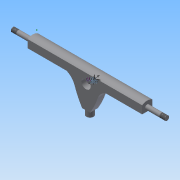
# Autodesk Inventor part: Truck
Saved by Autodesk Inventor 2015 (Build 190159000, 159)
## iProperties
Created: 2015-11-29
Part Number: Truck
Material: Generic
Document SubType Name: Modeling
Designer: JoshuaYuan
Density: 1 g/cm^3
Appearance: Default
Author: JoshuaYuan
Autodesk Inventor part; units mm, degrees
ref_plane "YZ Plane" through (0, 0, 0) normal (1, 0, 0) x (0, 1, 0)
ref_plane "XZ Plane" through (0, 0, 0) normal (0, 1, 0) x (-1, 0, 0)
ref_plane "XY Plane" through (0, 0, 0) normal (0, 0, 1) x (1, 0, 0)
sketch "Sketch1" plane through (0, 0, 0) normal (1, 0, 0) x (0, 1, 0)
  line L0 (-6.1783, -17.5347) -> (-20.1483, -17.5347)
  line L1 (-20.1483, -17.5347) -> (-20.1483, -35.5687)
  line L2 (-20.1483, -35.5687) -> (-6.1783, -35.5687)
  arc A0 (-6.1783, -35.5687) -> (-6.1783, -17.5347) centre (-19.1426, -26.5517) ccw
  point P0 (0, 0)
  dimension "d0" = 13.97
  dimension "d1" = 18.034
  constraints: 6 end point, 2 perpendicular, 2 point on circle, 1 centre point, 1 horizontal, 1 parallel
  measures "d0" distance of L1.end L2.end
  measures "d1" distance of L0.end L1.end
extrude "Truck Axle" add sketch "Sketch1" along normal blind 203.2
sketch "Sketch2" plane through (203.2, 0, 0) normal (1, 0, 0) x (0, 0, -1)
  circle A0 centre (26.5517, -13.1633) radius 3.9688
  line L0 (17.5347, -6.1783) -> (17.5347, -20.1483) projected
  line L1 (17.5347, -13.1633) -> (35.5687, -13.1633) construction
  line L2 (35.5687, -20.1483) -> (35.5687, -6.1783) projected
  point P0 (0, 0)
  point P1 (26.5517, -13.1633)
  dimension "d40" = 7.9375
  constraints: 3 midpoint, 2 end point, 1 centre point, 1 coincident
  measures "d40" diameter of A0
extrude "Axle" add sketch "Sketch2" along normal blind 34.925
ref_plane "Work Plane1" through (101.6, 0, 0) normal (1, 0, 0) x (0, 0, -1)
mirror "Other Axle" about plane through (101.6, 0, 0) normal (1, 0, 0) of "Axle"
ref_plane "Work Plane3" through (0, -20.1483, -26.5517) normal (0, 0, 1) x (1, 0, 0)
sketch "Sketch4" plane through (0, -20.1483, -26.5517) normal (0, 0, 1) x (1, 0, 0)
  line L0 (0, 0) -> (203.2, 0) projected
  line L1 (94.615, -45.72) -> (108.585, -45.72)
  line L2 (203.2, 13.97) -> (203.2, 0) projected
  line L3 (101.6, 0) -> (101.6, -45.72) construction
  line L4 (120.65, 0) -> (120.65, -24.9823)
  line L5 (120.65, -24.9823) -> (108.585, -45.72)
  line L6 (94.615, -45.72) -> (82.55, -24.9823)
  line L7 (82.55, -24.9823) -> (82.55, 0)
  point P0 (0, 20.1483)
  dimension "d25" = 13.97
  dimension "d49" = 45.72
  dimension "d50" = 38.1
  constraints: 12 end point, 2 equal length, 2 midpoint, 2 parallel, 2 point on line, 1 perpendicular, 1 vertical
  measures "d25" distance of L1.start L1.end
  measures "d49" distance between parallel lines of L0 L1
  measures "d50" distance between parallel lines of L7 L4
extrude "Pentagon" add sketch "Sketch4" along normal mid plane 14
fillet "Fillet1" radius 25.4 2 edges at (120.65, -20.1483, -26.5517) (82.55, -20.1483, -26.5517)
sketch "Sketch6" plane through (0, -20.1483, -33.5517) normal (0, 0, -1) x (-1, 0, 0)
  circle A0 centre (-101.6, -5.0143) radius 8.255
  circle A1 centre (-101.6, -5.0143) radius 12.7
  circle A2 centre (-101.6, -5.0143) radius 15
  point P0 (0, 20.1483)
  dimension "d54" = 16.51
  dimension "d56" = 25.4
  dimension "d57" = 30
  constraints: 3 centre point, 2 coincident
  measures "d54" diameter of A0
  measures "d56" diameter of A1
  measures "d57" diameter of A2
extrude "Inner hole" cut sketch "Sketch6" along normal mid plane 50.8 contours A0
sketch "Sketch10" plane through (94.615, -65.8683, -19.5517) normal (0, -1, 0) x (1, 0, 0)
  circle A0 centre (6.985, -7) radius 6.35
  line L0 (0, 0) -> (13.97, 0) projected
  line L1 (6.985, 0) -> (6.985, -14) construction
  line L2 (13.97, -14) -> (0, -14) projected
  point P0 (-94.615, 19.5517)
  dimension "d45" = 12.7
  constraints: 3 midpoint, 2 end point, 1 centre point, 1 coincident, 1 perpendicular
  measures "d45" diameter of A0
extrude "Ball joint" add sketch "Sketch10" along normal blind 10.16
fillet "Fillet3" [suppressed]
thread "Thread3" size "5/16-18 UNC" class "2A" standard "ANSI Unified Screw Threads" length 9.525
thread "Thread4" size "5/16-18 UNC" class "2A" standard "ANSI Unified Screw Threads" length 9.525
fillet "Fillet6" radius 127 2 edges at (120.6535, -45.1246, -26.5517) (82.5465, -45.1246, -26.5517)
ref_plane "Work Plane2" through (101.6, 0, 0) normal (1, 0, 0) x (0, 0, -1)
body "Solid1"
